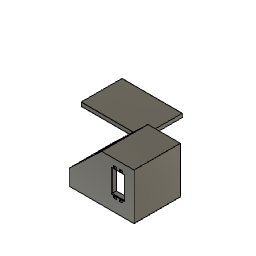
Modèle boitier v2 (Autodesk Fusion 360 design; units mm, degrees)
Autodesk Fusion 360 part; units mm, degrees
hole "Perçage1" at (-45, 20, 50) at (45, 20, 50) at (45, -20, 50) at (-45, -20, 50) direction (0, 0, -1) diameter 2.529 depth 12 tip angle 180
thread "Filetage1" [no effect]
sketch "Esquisse9" plane through (0, 0, 0) normal (0, 1, 0) x (1, 0, 0)
  line L0 (50, 0) -> (-20, 0)
  line L1 (-20, 0) -> (-20, -16.6667)
  line L2 (15, -50) -> (50, -50)
  line L3 (50, -50) -> (50, 0)
  line L4 (15, -50) -> (-20, -16.6667)
  point P0 (-20, -50)
  dimension "d52" = 70
  dimension "d53" = 50
  dimension "d54" = 35
  dimension "d55" = 33.3333
  constraint horizontal L0
  constraint vertical L1
  constraint horizontal L2
  constraint vertical L3
  constraint coincident P0 L2
  constraint coincident P0 L1
  measures "d52" distance of L0.start L0.end
  measures "d53" distance of L0.start L2.end
  measures "d54" distance of P0 L2.start
  measures "d55" distance of P0 L1.end
extrude "Extrusion7" add sketch "Esquisse9" along normal mid plane 50 makes body 1
shell "Coque1" thickness 5 removed faces 0 bodies 1
sketch "Esquisse11" plane through (0, 0, 0) normal (0, 0, 1) x (1, 0, 0)
  line L0 (50, 25) -> (-20, 25)
  line L1 (-20, 25) -> (-20, -25)
  line L2 (-20, -25) -> (50, -25)
  line L3 (50, -25) -> (50, 25)
  point P0 (-20, 25)
  point P1 (50, -25)
  constraint horizontal L0
  constraint vertical L1
  constraint horizontal L2
  constraint vertical L3
  constraint coincident P0 L0.end
  constraint coincident P1 L2.end
sketch "Esquisse12" plane through (-20, 0, 0) normal (-1, 0, 0) x (0, -1, 0)
  line L0 (-25, 0) -> (25, 0)
  line L1 (25, 0) -> (25, 16.6667)
  line L2 (25, 16.6667) -> (-25, 16.6667)
  line L3 (-25, 16.6667) -> (-25, 0)
  line L4 (25, 0) -> (-25, 0)
  line L5 (-25, 0) -> (25, 0)
  line L6 (0, 0) -> (0, 5)
  line L7 (-22.5, 2.5) -> (22.5, 2.5)
  line L8 (22.5, 2.5) -> (22.5, 7.5)
  line L9 (22.5, 7.5) -> (-22.5, 7.5)
  line L10 (-22.5, 7.5) -> (-22.5, 2.5)
  line L11 (-22.5, 2.5) -> (22.5, 7.5) construction
  line L12 (22.5, 2.5) -> (-22.5, 7.5) construction
  line L13 (-20, -2.5) -> (20, -2.5)
  line L14 (20, -2.5) -> (20, 2.5)
  line L15 (20, 2.5) -> (-20, 2.5)
  line L16 (-20, 2.5) -> (-20, -2.5)
  line L17 (-20, -2.5) -> (20, 2.5) construction
  line L18 (20, -2.5) -> (-20, 2.5) construction
  point P0 (-25, 0)
  point P1 (0, 5)
  dimension "d59" = 45
  dimension "d60" = 5
  dimension "d61" = 5
  dimension "d62" = 40
  dimension "d63" = 5
  constraint coincident L0.end L1.start
  constraint coincident P0 L0.start
  constraint midpoint L6.start L5
  constraint parallel L1 L6
  constraint coincident L6.start origin
  constraint horizontal L7
  constraint perpendicular L7 L8
  constraint parallel L7 L9
  constraint parallel L8 L10
  constraint coincident L11 P1
  constraint coincident L12 P1
  constraint coincident P1 L6.end
  constraint horizontal L13
  constraint perpendicular L13 L14
  constraint parallel L13 L15
  constraint parallel L14 L16
  constraint coincident L17 L6.start
  constraint coincident L18 L6.start
  measures "d59" distance of L8.end L9.end
  measures "d60" distance of L7.end L8.end
  measures "d61" distance of L6.start P1
  measures "d62" distance of L14.end L15.end
  measures "d63" distance of L13.end L14.end
extrude "Extrusion8" cut sketch "Esquisse12" against normal blind 65 contours L0 L4 L5 L6 L7 L15 L16 | L0 L4 L5 L6 L7 L14 L15 | L7 L8 L9 L10 L15 bodies 1
sketch "Esquisse13" plane through (-20, 0, 0) normal (-1, 0, 0) x (0, -1, 0)
  line L0 (-53, 3) -> (-97, 3)
  line L1 (-97, 3) -> (-97, 7)
  line L2 (-97, 7) -> (-53, 7)
  line L3 (-53, 7) -> (-53, 3)
  dimension "d66" = 44
  dimension "d67" = 4
  constraint horizontal L0
  constraint vertical L1
  constraint horizontal L2
  constraint vertical L3
  measures "d66" distance of L0.start L0.end
  measures "d67" distance of L0.start L2.end
extrude "Extrusion9" add sketch "Esquisse13" along normal blind 65 separate body makes body 2
sketch "Esquisse14" plane through (-17.8359, 0, 18.7277) normal (-0.689655, 0, 0.724138) x (0, -1, 0)
  line L0 (-25, -2.9885) -> (25, -2.9885)
  line L1 (25, -2.9885) -> (25, 45.3448)
  line L2 (25, 45.3448) -> (-25, 45.3448)
  line L3 (-25, 45.3448) -> (-25, -2.9885)
  line L4 (0, 45.3448) -> (0, 28.3448)
  line L5 (12.5, 35.3448) -> (-12.5, 35.3448)
  line L6 (-13, 34.8448) -> (-13, 21.8448)
  line L7 (-12.5, 21.3448) -> (12.5, 21.3448)
  line L8 (13, 21.8448) -> (13, 34.8448)
  line L9 (13, 35.3448) -> (-13, 21.3448) construction
  line L10 (-13, 35.3448) -> (13, 21.3448) construction
  arc A0 (-12.5, 35.3448) -> (-13, 34.8448) centre (-12.5, 34.8448) ccw
  arc A1 (13, 34.8448) -> (12.5, 35.3448) centre (12.5, 34.8448) ccw
  arc A2 (12.5, 21.3448) -> (13, 21.8448) centre (12.5, 21.8448) ccw
  arc A3 (-13, 21.8448) -> (-12.5, 21.3448) centre (-12.5, 21.8448) ccw
  point P0 (0, 45.3448)
  point P1 (0, 28.3448)
  dimension "d72" = 26
  dimension "d73" = 14
  dimension "d74" = 17
  dimension "d75" = 0.5
  dimension "d76" = 0.5
  dimension "d77" = 0.5
  dimension "d78" = 0.5
  constraint midpoint L2 P0
  constraint vertical L4
  constraint coincident P0 L4.start
  constraint horizontal L5
  constraint perpendicular L5 L6
  constraint parallel L5 L7
  constraint parallel L6 L8
  constraint coincident L9 P1
  constraint coincident L10 P1
  constraint coincident P1 L4.end
  constraint coincident L10.start L6
  constraint coincident L10.start L5
  constraint tangent L6 A0
  constraint tangent L5 A0
  constraint coincident L9.start L5
  constraint coincident L9.start L8
  constraint tangent L5 A1
  constraint tangent L8 A1
  constraint coincident L10.end L8
  constraint coincident L10.end L7
  constraint tangent L8 A2
  constraint tangent L7 A2
  constraint coincident L9.end L6
  constraint coincident L9.end L7
  constraint tangent L6 A3
  constraint tangent L7 A3
  measures "d72" distance of L9.end L10.end
  measures "d73" distance of L10.start L9.end
  measures "d74" distance of P0 P1
  measures "d75" radius of A0
  measures "d76" radius of A1
  measures "d77" radius of A2
  measures "d78" radius of A3
extrude "Extrusion10" cut sketch "Esquisse14" against normal blind 5 contours L5 L6 L7 L8 A0 A1 A2 A3 bodies 1
sketch "Esquisse15" plane through (0, -25, 0) normal (0, -1, 0) x (1, 0, 0)
  line L0 (50, 0) -> (50, 50)
  line L1 (50, 50) -> (15, 50)
  line L2 (15, 50) -> (-20, 16.6667)
  line L3 (-20, 16.6667) -> (-20, 0)
  line L4 (-20, 0) -> (50, 0)
  line L5 (39, 40) -> (26, 40)
  line L6 (26, 40) -> (26, 16)
  line L7 (26, 16) -> (39, 16)
  line L8 (39, 16) -> (39, 40)
  line L9 (39, 40) -> (26, 16) construction
  line L10 (26, 40) -> (39, 16) construction
  line L11 (32.5, 50) -> (32.5, 28)
  line L12 (35.75, 42) -> (29.25, 42)
  line L13 (29.25, 42) -> (29.25, 14)
  line L14 (29.25, 14) -> (35.75, 14)
  line L15 (35.75, 14) -> (35.75, 42)
  line L16 (35.75, 42) -> (29.25, 14) construction
  line L17 (29.25, 42) -> (35.75, 14) construction
  point P0 (32.5, 50)
  point P1 (32.5, 28)
  point P2 (32.5, 28)
  dimension "d82" = 13
  dimension "d83" = 24
  dimension "d84" = 22
  dimension "d86" = 6.5
  dimension "d87" = 28
  constraint midpoint L1 P0
  constraint horizontal L5
  constraint perpendicular L5 L6
  constraint parallel L5 L7
  constraint parallel L6 L8
  constraint coincident L9 P2
  constraint coincident L10 P2
  constraint coincident P0 L11.start
  constraint parallel L0 L11
  constraint coincident P2 P1
  constraint horizontal L12
  constraint perpendicular L12 L13
  constraint parallel L12 L14
  constraint parallel L13 L15
  constraint coincident L16 P2
  constraint coincident L17 P2
  measures "d82" distance of L6.end L7.end
  measures "d83" distance of L5.end L6.end
  measures "d84" distance of P0 P2
  measures "d86" distance of L13.end L14.end
  measures "d87" distance of L12.end L13.end
sketch "Esquisse16" plane through (32.5, -25, 28) normal (0, -1, 0) x (1, 0, 0)
  line L0 (4.75, 15) -> (1.75, 15)
  line L1 (1.75, 15) -> (1.75, 13)
  line L2 (1.75, 13) -> (4.75, 13)
  line L3 (4.75, 13) -> (4.75, 15)
  line L4 (4.75, 15) -> (1.75, 13) construction
  line L5 (1.75, 15) -> (4.75, 13) construction
  line L6 (-1.75, 13) -> (-1.75, 15)
  line L7 (-1.75, 15) -> (-4.75, 13) construction
  line L8 (-1.75, 15) -> (-4.75, 15)
  line L9 (-4.75, 15) -> (-4.75, 13)
  line L10 (-4.75, 15) -> (-1.75, 13) construction
  line L11 (-4.75, 13) -> (-1.75, 13)
  line L12 (-1.75, -15) -> (-1.75, -13)
  line L13 (-1.75, -13) -> (-4.75, -15) construction
  line L14 (-1.75, -13) -> (-4.75, -13)
  line L15 (-4.75, -13) -> (-4.75, -15)
  line L16 (-4.75, -13) -> (-1.75, -15) construction
  line L17 (-4.75, -15) -> (-1.75, -15)
  line L18 (4.75, -15) -> (4.75, -13)
  line L19 (4.75, -13) -> (1.75, -15) construction
  line L20 (4.75, -13) -> (1.75, -13)
  line L21 (1.75, -13) -> (1.75, -15)
  line L22 (1.75, -13) -> (4.75, -15) construction
  line L23 (1.75, -15) -> (4.75, -15)
  point P0 (3.25, 14)
  point P1 (-3.25, 14)
  point P2 (-3.25, -14)
  point P3 (3.25, -14)
  point P4 (3.25, 14)
  point P5 (-3.25, 14)
  point P6 (-3.25, -14)
  point P7 (3.25, -14)
  dimension "d88" = 3
  dimension "d89" = 2
  dimension "d90" = 3
  dimension "d91" = 2
  dimension "d92" = 3
  dimension "d93" = 2
  dimension "d94" = 3
  dimension "d95" = 2
  constraint horizontal L0
  constraint perpendicular L0 L1
  constraint parallel L0 L2
  constraint parallel L1 L3
  constraint coincident L4 P4
  constraint coincident L5 P4
  constraint horizontal L8
  constraint perpendicular L8 L9
  constraint parallel L8 L11
  constraint parallel L6 L9
  constraint coincident P5 L7
  constraint coincident P5 L10
  constraint horizontal L14
  constraint perpendicular L14 L15
  constraint parallel L14 L17
  constraint parallel L12 L15
  constraint coincident P6 L13
  constraint coincident P6 L16
  constraint horizontal L20
  constraint perpendicular L20 L21
  constraint parallel L20 L23
  constraint parallel L18 L21
  constraint coincident P7 L19
  constraint coincident P7 L22
  constraint coincident P4 P0
  constraint coincident P5 P1
  constraint coincident P6 P2
  constraint coincident P7 P3
  measures "d88" distance of L1.end L2.end
  measures "d89" distance of L0.end L1.end
  measures "d90" distance of L7.end L6.start
  measures "d91" distance of L7.end L8.end
  measures "d92" distance of L13.end L12.start
  measures "d93" distance of L13.end L14.end
  measures "d94" distance of L19.end L18.start
  measures "d95" distance of L19.end L20.end
extrude "Extrusion11" cut sketch "Esquisse15" sketch "Esquisse16" against normal blind 5 contours L5 L7 L8 L15 | L5 L7 L13 L15 | L5 L6 L7 L13 of sketch 2 bodies 1
chamfer "Chanfrein1" distance 1.6667 distance2 5 8 edges at (7.7586, 0, 43.1034) (7.6526, -12.8536, 43.0025) (2.6897, -13, 38.2759) (-2.2733, -12.8536, 33.5493) (-2.3793, 0, 33.4483) (-2.2733, 12.8536, 33.5493) (2.6897, 13, 38.2759) (7.6526, 12.8536, 43.0025) measured on face at (-14.1264, -4.1667, 22.2605) measured on face at (-14.1264, -4.1667, 22.2605) measured on face at (-14.1264, -4.1667, 22.2605) measured on face at (-14.1264, -4.1667, 22.2605) measured on face at (-14.1264, -4.1667, 22.2605) measured on face at (-14.1264, -4.1667, 22.2605) measured on face at (-14.1264, -4.1667, 22.2605) measured on face at (-14.1264, -4.1667, 22.2605) on bodies 1
chamfer "Chanfrein2" distance 0.5 distance2 0.5 4 edges at (26, -25, 28) (32.5, -25, 40) (39, -25, 28) (32.5, -25, 16) measured on face at (7, -25, 27.5556) measured on face at (7, -25, 27.5556) measured on face at (7, -25, 27.5556) measured on face at (7, -25, 27.5556) on bodies 1
equation "longueur = 70 mm"
equation "Largeur = 50 mm"
equation "hauteur = 50 mm"
equation "epaisseur = 5 mm"
equation "rayon_exterieur = 5 mm"
equation "visse_longueur = 12 mm"
equation "d28 = visse_longueur"
equation "visse_tete_hauteur = 3 mm"
equation "visse_tete_diametre = 5 mm"
equation "visse_diametre = 3 mm"
equation "ecran_longueur = 26 mm"
equation "ecran_largeur = 14 mm"
equation "drapeau_largeur = 13 mm"
equation "drapeau_longueur = 24 mm"
equation "d52 = longueur"
equation "d53 = hauteur"
equation "d54 = longueur / 2"
equation "d55 = hauteur / 1.5"
equation "d58 = epaisseur"
equation "d59 = Largeur - epaisseur"
equation "d60 = epaisseur"
equation "d61 = epaisseur"
equation "d62 = Largeur - epaisseur * 2"
equation "d63 = epaisseur"
equation "d64 = -( longueur - epaisseur )"
equation "d66 = Largeur - epaisseur - jeu"
equation "d67 = epaisseur - jeu"
equation "jeu = 1 mm"
equation "d69 = longueur - epaisseur"
equation "ecran_decallage = 10 mm"
equation "d72 = ecran_longueur"
equation "d73 = ecran_largeur"
equation "d74 = ecran_decallage + ecran_largeur / 2"
equation "d79 = -epaisseur"
equation "drapeau_decallage = 10 mm"
equation "d82 = drapeau_largeur"
equation "d83 = drapeau_longueur"
equation "d84 = drapeau_decallage + drapeau_longueur / 2"
equation "drapeau_attache_longueur = 28 mm"
equation "d86 = drapeau_largeur / 2"
equation "d87 = drapeau_attache_longueur"
equation "d96 = -epaisseur"
equation "d98 = epaisseur / 3"
equation "d99 = epaisseur"
